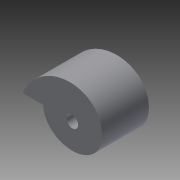
# Autodesk Inventor part: cam 2
Saved by Autodesk Inventor 2014 (Build 180170000, 170)
## iProperties
Created: 2014-05-19
Part Number: cam 2
Material: Generic
Document SubType Name: Modeling
Designer: jyesowitz
Density: 1 g/cm^3
Appearance: Default
Author: jyesowitz
Autodesk Inventor part; units mm, degrees
ref_plane "YZ Plane" through (0, 0, 0) normal (1, 0, 0) x (0, 1, 0)
ref_plane "XZ Plane" through (0, 0, 0) normal (0, 1, 0) x (-1, 0, 0)
ref_plane "XY Plane" through (0, 0, 0) normal (0, 0, 1) x (1, 0, 0)
sketch "Sketch1" plane through (0, 0, 0) normal (0, 0, 1) x (1, 0, 0)
  ellipse E0 centre (0, 0) end of major axis (31.369, 0) minor radius 27.2774 (-31.369, 0) -> (30.4208, -6.656) ccw
  line L0 (30.4208, -6.656) -> (41.3005, 30.9432) construction
  line L1 (41.3005, 30.9432) -> (0, 54.7437) construction
  line L2 (0, 54.7437) -> (-41.2495, 30.9545) construction
  line L3 (-41.2495, 30.9545) -> (-53.8557, 0) construction
  spline S0 degree 4 poles (30.4208, -6.656) (41.3005, 30.9432) (0, 54.7437) (-41.2495, 30.9545) (-53.8557, 0) knots 1 1 1 1 1 2 2 2 2 2
  line L4 (-53.8557, 0) -> (-31.369, 0)
  circle A0 centre (0, 0) radius 6.35
  dimension "d49" = 31.369
  dimension "d16" = 0
  dimension "d18" = 53.8557
  dimension "d19" = 22.4867
  dimension "d29" = 54.7437
  dimension "d30" = 47.6177
  dimension "d31" = 33.423
  dimension "d32" = 47.6676
  dimension "d33" = 39.1416
  dimension "d43" = 120.074
  dimension "d50" = 12.7
  constraints: 2 end point, 1 centre point, 1 coincident, 1 horizontal, 8 other
  measures "d16" distance of point (0, 0) point (0, 0)
  measures "d18" distance of point (0, 0) L3.end
  measures "d19" distance of L3.end L4.end
  measures "d29" distance of L1.end point (0, 0)
  measures "d30" distance of L1.end L2.end
  measures "d31" distance of L2.end L3.end
  measures "d32" distance of L0.end L1.end
  measures "d33" distance of L0.start L0.end
  measures "d43" angle of L2 L1
  measures "d50" diameter of A0
extrude "Extrusion1" add sketch "Sketch1" against normal blind 50.8
body "Solid1"
